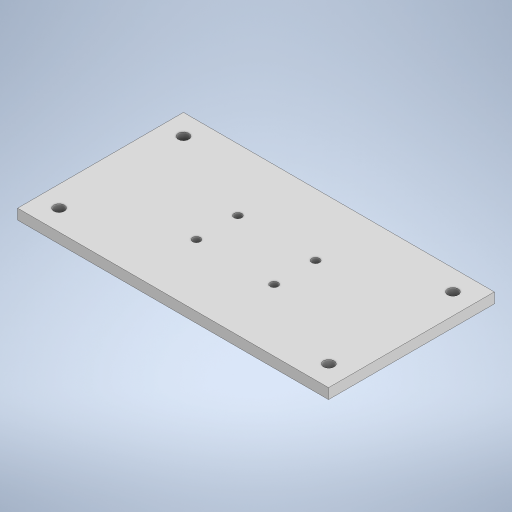
# Autodesk Inventor part: SequenceMachine_ManifoldPlate
Saved by Autodesk Inventor 2023 (Build 270158000, 158)
## iProperties
Created: 2022-07-18
Part Number: SequenceMachine_ManifoldPlate
Material: Generic
Document SubType Name: Modeling
Designer: devon
Density: 1 g/cm^3
Appearance: Default
Author: devon
Autodesk Inventor part; units mm, degrees
ref_plane "YZ Plane" through (0, 0, 0) normal (1, 0, 0) x (0, 1, 0)
ref_plane "XZ Plane" through (0, 0, 0) normal (0, 1, 0) x (-1, 0, 0)
ref_plane "XY Plane" through (0, 0, 0) normal (0, 0, 1) x (1, 0, 0)
sketch "Sketch1" plane through (0, 0, 0) normal (0, 1, 0) x (-1, 0, 0)
  line L0 (95.25, 50.8) -> (-95.25, 50.8)
  line L1 (-95.25, 50.8) -> (-95.25, -50.8)
  line L2 (-95.25, -50.8) -> (95.25, -50.8)
  line L3 (95.25, -50.8) -> (95.25, 50.8)
  line L4 (95.25, 50.8) -> (-95.25, -50.8) construction
  line L5 (-95.25, 50.8) -> (95.25, -50.8) construction
  circle A0 centre (82.55, -38.1) radius 3.302
  circle A1 centre (-82.55, -38.1) radius 3.302
  circle A2 centre (-82.7024, 38.1) radius 3.302
  circle A3 centre (82.55, 38.1) radius 3.302
  line L6 (40.9111, -12.7) -> (-47.9889, -12.7) construction
  line L7 (40.9111, 12.7) -> (-47.9889, 12.7) construction
  circle A4 centre (23.8125, -12.7) radius 2.413
  circle A5 centre (-23.8125, -12.7) radius 2.413
  circle A6 centre (23.8125, 12.7) radius 2.413
  circle A7 centre (-23.8125, 12.7) radius 2.413
  point P0 (0, 0)
  dimension "d0" = 190.5
  dimension "d1" = 101.6
  dimension "d2" = 6.604
  dimension "d3" = 12.7
  dimension "d4" = 12.7
  dimension "d5" = 6.604
  dimension "d6" = 12.7
  dimension "d7" = 6.604
  dimension "d8" = 12.7
  dimension "d9" = 6.604
  dimension "d10" = 88.9
  dimension "d11" = 88.9
  dimension "d12" = 25.4
  dimension "d13" = 12.7
  dimension "d14" = 4.826
  dimension "d15" = 4.826
  dimension "d16" = 47.625
  dimension "d17" = 23.8125
  dimension "d18" = 4.826
  dimension "d19" = 4.826
  dimension "d22" = 12.7
  dimension "d23" = 12.7
  constraints: 16 end point, 8 centre point, 4 point on line, 3 horizontal, 2 midpoint, 2 parallel, 1 perpendicular
  measures "d0" distance of L1.end L2.end
  measures "d1" distance of L0.end L1.end
  measures "d2" diameter of A0
  measures "d3" distance from line of L2 A0.centre
  measures "d4" distance from line of L3 A0.centre
  measures "d5" diameter of A1
  measures "d6" distance from line of L1 A1.centre
  measures "d7" diameter of A2
  measures "d8" distance from line of L0 A2.centre
  measures "d9" diameter of A3
  measures "d10" distance of L6.start L6.end
  measures "d11" distance of L7.start L7.end
  measures "d12" distance between parallel lines of L7 L6
  measures "d13" distance from line of point (0, 0) L6
  measures "d14" diameter of A4
  measures "d15" diameter of A5
  measures "d16" distance of A5.centre A4.centre
  measures "d17" horizontal distance of point (0, 0) A4.centre
  measures "d18" diameter of A6
  measures "d19" diameter of A7
  measures "d22" distance from line of L0 A3.centre
  measures "d23" distance from line of L3 A3.centre
extrude "Extrusion1" add sketch "Sketch1" along normal blind 6.35
equation "\"d13\" = 0.5 * d12"
equation "\"d17\" = 0.5 * d16"
body "Solid1"
